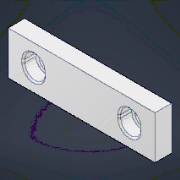
# Autodesk Inventor part: JawDualSided
Saved by Autodesk Inventor 2024.3 (Build 283343000, 343)
## iProperties
IsCustomPart: 1
Created: 2024-02-05
Part Number: JawDualSided
Material: Aluminum 6061
Document SubType Name: Modeling
Designer: fablabadmin
Language: en-US
Size Designation: JawDualSided-Aluminum 6061
Categories: <MemberInstance><Categories><Category DisplayName="CAM_JAWS" InternalName="a455355c-d78b-4130-92af-7f17fb1dc89c" Mnemonic="CAM_JAWS"/><Category DisplayName="DataType" InternalName="23b78d0f-2648-40c6-8793-ca6db495c9e8" Mnemonic="DATATYPE"><CategoryParameter DisplayName="DisplayName" InternalName="05415f3d-3907-474b-a020-eb9d644f4cf3" Mnemonic="DISPLAYNAME"/><CategoryParameter DisplayName="Standard" InternalName="0c0a119c-1e12-4c84-803f-101930972f5e" Mnemonic="STANDARD"/><CategoryParameter DisplayName="Description" InternalName="13903e3d-64b1-4950-80da-f627842ea37f" Mnemonic="DESCRIPTION"/><CategoryParameter DisplayName="Designation" InternalName="2675968c-4ce5-49e0-a4f5-552d29089031" Mnemonic="DESIGNATION"/><CategoryParameter DisplayName="Default Row" InternalName="2af9ec52-faaa-4026-b378-f9fa4afca842" Mnemonic="DEFAULTROW"/><CategoryParameter DisplayName="Folder Name" InternalName="3f06958e-8713-4116-9be7-ed6184ecc97b" Mnemonic="FOLDERNAME"/><CategoryParameter DisplayName="Revision Guid" InternalName="45a75005-10b1-4dfc-8d6d-dfe629f0b93c" Mnemonic="REVISIONGUID"/><CategoryParameter DisplayName="FileName" InternalName="8b46a4cc-9585-4fed-90c3-899f57e09a73" Mnemonic="FILENAME"/><CategoryParameter DisplayName="StdsOrg" InternalName="8f5914e1-4693-403f-8ab5-d37768198c9d" Mnemonic="STDSORG"/><CategoryParameter DisplayName="Family Version" InternalName="914462f6-6e19-4b14-ba84-155b9680b1d0" Mnemonic="FAMILYREVISION"/><CategoryParameter DisplayName="Standard Revision" InternalName="91d5a463-65c2-4fde-b823-3b7fea5e8e17" Mnemonic="STANDARDREVISION"/><CategoryParameter DisplayName="Member Revision" InternalName="a65d44b9-392f-4f4f-857b-e4b3d54996fe" Mnemonic="MEMBERREVISION"/><CategoryParameter DisplayName="ClipFormat" InternalName="bc51e27b-3422-4e78-93ef-cec197ddf230" Mnemonic="CLIPFORMAT"/><CategoryParameter DisplayName="Manufacturer" InternalName="cd6c7a72-a28a-4e50-99a9-2c7f4e13e5ad" Mnemonic="MANUFACTURER"/><CategoryParameter DisplayName="InternalName" InternalName="cf1d0246-76d9-4b4a-8305-fa0409afb5c1" Mnemonic="INTERNALNAME"/><CategoryParameter DisplayName="IsMetric" InternalName="e2385c5b-1ea4-4823-96a8-8de651266ec3" Mnemonic="ISMETRIC"/><Category DisplayName="Part" InternalName="c0e0b642-3bcb-4cc8-9e80-f96d35c4afa4" Mnemonic="PART"><CategoryParameter DisplayName="Part Number" InternalName="016b6077-bfbe-49bd-92c9-d8d59c39c941" Mnemonic="PARTNUMBER"/><CategoryParameter DisplayName="Stock Number" InternalName="4dba7c1c-e26c-444e-836c-b08b433409a8" Mnemonic="STOCKNUMBER"/><CategoryParameter DisplayName="Material Key" InternalName="5c9a8adb-dd2b-4535-b97f-0a94a95fe41f" Mnemonic="MATERIALKEY"/><CategoryParameter DisplayName="Material" InternalName="818a152a-d3c3-49ca-80ee-df7d91421b8e" Mnemonic="MATERIAL"/></Category></Category></Categories><FamilyTemplate Id="DualSidedJaw"><FamilyTemplateParameters><FamilyTemplateParameter ObjectType="kPartComponentDefinitionObject" ValueType="xs:string" Id="11" SubObjectId="Material"/><FamilyTemplateParameter ObjectType="kPropertyObject" ValueType="xs:string" Id="18" ObjectReferenceKey="{32853F0F-3444-11d1-9E93-0060B03C1CA6}" SubObjectId="5"/><FamilyTemplateParameter ObjectType="kPropertyObject" ValueType="xs:string" Id="19" ObjectReferenceKey="{32853F0F-3444-11d1-9E93-0060B03C1CA6}" SubObjectId="52"/></FamilyTemplateParameters></FamilyTemplate><CategoryParameterMap><ParamToTemplateMap><ParamToTemplate CategoryParameter="//CategoryParameter[@InternalName='cf1d0246-76d9-4b4a-8305-fa0409afb5c1']" ConstantValue="43a365f2-93b3-4b52-b820-3dbb13a23e22"/><ParamToTemplate CategoryParameter="//CategoryParameter[@InternalName='45a75005-10b1-4dfc-8d6d-dfe629f0b93c']" ConstantValue="9f47d84c-379b-4d57-88d0-f6fbd2db50da"/><ParamToTemplate CategoryParameter="//CategoryParameter[@InternalName='3f06958e-8713-4116-9be7-ed6184ecc97b']" ConstantValue="DualSidedJaw"/><ParamToTemplate CategoryParameter="//CategoryParameter[@InternalName='8f5914e1-4693-403f-8ab5-d37768198c9d']" TemplateParameter="5"/><ParamToTemplate CategoryParameter="//CategoryParameter[@InternalName='0c0a119c-1e12-4c84-803f-101930972f5e']" TemplateParameter="6"/><ParamToTemplate CategoryParameter="//CategoryParameter[@InternalName='91d5a463-65c2-4fde-b823-3b7fea5e8e17']" TemplateParameter="7"/><ParamToTemplate CategoryParameter="//CategoryParameter[@InternalName='cd6c7a72-a28a-4e50-99a9-2c7f4e13e5ad']" TemplateParameter="8"/><ParamToTemplate CategoryParameter="//CategoryParameter[@InternalName='13903e3d-64b1-4950-80da-f627842ea37f']" TemplateParameter="10"/><ParamToTemplate CategoryParameter="//CategoryParameter[@InternalName='05415f3d-3907-474b-a020-eb9d644f4cf3']" ConstantValue="JawDual"/><ParamToTemplate CategoryParameter="//CategoryParameter[@InternalName='914462f6-6e19-4b14-ba84-155b9680b1d0']" ConstantValue="11"/><ParamToTemplate CategoryParameter="//CategoryParameter[@InternalName='bc51e27b-3422-4e78-93ef-cec197ddf230']" ConstantValue="CF_INVENTOR.STDPARTS"/><ParamToTemplate CategoryParameter="//CategoryParameter[@InternalName='e2385c5b-1ea4-4823-96a8-8de651266ec3']" ConstantValue="true"/><ParamToTemplate CategoryParameter="//CategoryParameter[@InternalName='2af9ec52-faaa-4026-b378-f9fa4afca842']" ConstantValue="1"/><ParamToTemplate CategoryParameter="//CategoryParameter[@InternalName='8b46a4cc-9585-4fed-90c3-899f57e09a73']" ConstantValue="JawDualSided-Aluminum 6061"/><ParamToTemplate CategoryParameter="//CategoryParameter[@InternalName='a65d44b9-392f-4f4f-857b-e4b3d54996fe']" ConstantValue="5ccd6349-9766-45ff-ba35-29068830a0fb"/><ParamToTemplate CategoryParameter="//CategoryParameter[@InternalName='a65d44b9-392f-4f4f-857b-e4b3d54996fe']" ConstantValue="5ccd6349-9766-45ff-ba35-29068830a0fb"/><ParamToTemplate CategoryParameter="//CategoryParameter[@InternalName='2675968c-4ce5-49e0-a4f5-552d29089031']" TemplateParameter="19"/><ParamToTemplate CategoryParameter="//CategoryParameter[@InternalName='818a152a-d3c3-49ca-80ee-df7d91421b8e']" TemplateParameter="11"/><ParamToTemplate CategoryParameter="//CategoryParameter[@InternalName='016b6077-bfbe-49bd-92c9-d8d59c39c941']" TemplateParameter="18"/></ParamToTemplateMap></CategoryParameterMap></MemberInstance>
Density: 2.7 g/cm^3
Appearance: Aluminum - Flat
Author: fablabadmin
Autodesk Inventor part; units mm, degrees
ref_plane "YZ Plane" through (0, 0, 0) normal (1, 0, 0) x (0, 1, 0)
ref_plane "XZ Plane" through (0, 0, 0) normal (0, 1, 0) x (-1, 0, 0)
ref_plane "XY Plane" through (0, 0, 0) normal (0, 0, 1) x (1, 0, 0)
sketch "Sketch1" plane through (0, 0, 0) normal (0, 0, 1) x (1, 0, 0)
  line L0 (-105.56, 0) -> (105.56, 0) construction
  line L1 (0, -31.15) -> (0, 31.15) construction
  line L2 (-75.5, 22.25) -> (75.5, 22.25)
  line L3 (75.5, 22.25) -> (75.5, -22.25)
  line L4 (75.5, -22.25) -> (-75.5, -22.25)
  line L5 (-75.5, -22.25) -> (-75.5, 22.25)
  line L6 (-49.21, 1.55) -> (-49.21, -1.55) construction
  line L7 (-56.21, 1.55) -> (-56.21, -1.55)
  line L8 (-42.21, -1.55) -> (-42.21, 1.55)
  arc A0 (-42.21, 1.55) -> (-56.21, 1.55) centre (-49.21, 1.55) ccw
  arc A1 (-56.21, -1.55) -> (-42.21, -1.55) centre (-49.21, -1.55) ccw
  line L9 (49.21, 1.55) -> (49.21, -1.55) construction
  line L10 (56.21, 1.55) -> (56.21, -1.55)
  line L11 (42.21, -1.55) -> (42.21, 1.55)
  arc A2 (56.21, 1.55) -> (42.21, 1.55) centre (49.21, 1.55) ccw
  arc A3 (42.21, -1.55) -> (56.21, -1.55) centre (49.21, -1.55) ccw
  line L12 (-49.21, 1.55) -> (-49.21, -1.55) construction
  line L13 (-59.71, 1.55) -> (-59.71, -1.55)
  line L14 (-38.71, -1.55) -> (-38.71, 1.55)
  arc A4 (-38.71, 1.55) -> (-59.71, 1.55) centre (-49.21, 1.55) ccw
  arc A5 (-59.71, -1.55) -> (-38.71, -1.55) centre (-49.21, -1.55) ccw
  line L15 (59.71, 1.55) -> (59.71, -1.55)
  line L16 (38.71, -1.55) -> (38.71, 1.55)
  arc A6 (59.71, 1.55) -> (38.71, 1.55) centre (49.21, 1.55) ccw
  arc A7 (38.71, -1.55) -> (59.71, -1.55) centre (49.21, -1.55) ccw
  point P0 (0, 0)
  point P1 (-49.21, 0)
  point P2 (49.21, 0)
  point P3 (-49.21, 0)
  dimension "d0" = 44.5
  dimension "d1" = 151
  dimension "d26" = 14
  dimension "d27" = 20.7
  dimension "d28" = 98.42
  dimension "d29" = 21
  dimension "d30" = 1.55
  constraints: 36 end point, 16 point on circle, 11 symmetric about line, 8 centre point, 8 tangent, 5 equal length, 2 midpoint, 1 horizontal, 1 perpendicular, 1 point on line, 1 vertical, 6 other
  measures "d0" distance of L2.end L3.end
  measures "d1" distance of L2.start L2.end
  measures "d26" distance between parallel lines of L8 L7
  measures "d27" distance from line of L4 L6.end
  measures "d28" distance between parallel lines of L9 L6
  measures "d29" distance between parallel lines of L13 L14
  measures "d30" distance from line of L0 L6.end
extrude "Extrusion1" add sketch "Sketch1" against normal blind 18 contours L2 L3 L4 L5 | A0 L8 A1 L7 | L10 A3 L11 A2 | A4 L14 A5 L13 | L15 A7 L16 A6
extrude "Extrusion2" cut sketch "Sketch1" against normal through all contours A0 L8 A1 L7 | L10 A3 L11 A2
extrude "Extrusion3" cut sketch "Sketch1" against normal blind 12.78 contours L10 A3 L11 A2 | A4 L14 A5 L13 | L15 A7 L16 A6
chamfer "Chamfer3" distance 1 angle 45 4 edges at (0, 22.25, -18) (-75.5, 0, -18) (0, -22.25, -18) (75.5, 0, -18)
chamfer "Chamfer4" distance 1.5 angle 45 8 edges at (-49.21, 12.05, 0) (-38.71, 0, 0) (-49.21, -12.05, 0) (-59.71, 0, 0) (49.21, 12.05, 0) (59.71, 0, 0) (49.21, -12.05, 0) (38.71, 0, 0)
chamfer "Chamfer5" distance 0.5 angle 45 8 edges at (-49.21, 8.55, -18) (-56.21, 0, -18) (-49.21, -8.55, -18) (-42.21, 0, -18) (49.21, -8.55, -18) (56.21, 0, -18) (49.21, 8.55, -18) (42.21, 0, -18)
sketch "Sketch2" plane through (-75.5, 22.25, 0) normal (0, 1, 0) x (1, 0, 0)
  line L0 (0, 17) -> (151, 17) construction
  line L1 (0, 0) -> (0, 17) construction
  line L2 (151, 0) -> (0, 0) projected
  line L3 (151, 0) -> (151, 17) construction
  line L4 (75.5, 21.6) -> (75.5, -3.6) construction
  circle A0 centre (75.5, -32.1751) radius 47.5 construction
  line L5 (150, 18) -> (1, 18) projected
  line L6 (58.5, 18) -> (40.5, 0)
  line L7 (92.5, 18) -> (110.5, 0)
  line L8 (14.29, 0) -> (38.29, 0) projected
  line L9 (33, 0) -> (51, 18)
  line L10 (118, 0) -> (100, 18)
  circle A1 centre (75.5, -28.2107) radius 50 construction
  line L11 (56.5, 16) -> (94.5, 16)
  dimension "d54" = 95
  dimension "d57" = 45
  dimension "d59" = 70
  dimension "d60" = 45
  dimension "d61" = 85
  dimension "d62" = 100
  dimension "d68" = 2
  constraints: 10 end point, 8 point on line, 4 symmetric about line, 2 centre point, 2 tangent, 1 parallel
  measures "d54" diameter of A0
  measures "d57" angle of L2 L6
  measures "d59" distance of L7.end L6.end
  measures "d60" angle of L2 L9
  measures "d61" distance of L10.start L9.start
  measures "d62" diameter of A1
  measures "d68" distance between parallel lines of L5 L11
extrude "Extrusion6" cut sketch "Sketch2" against normal blind 35 contours L2 L6 L11 L7
extrude "Extrusion7" cut sketch "Sketch2" against normal blind 6 contours L2 L7 L5 L10 | L2 L9 L5 L6 | L11 L6 L5 L7
fillet "Fillet1" radius 10 2 edges at (-19, 1.75, -16) (19, 1.75, -16)
equation "\"d0\" = jawH"
equation "\"d1\" = jawW"
equation "\"d4\" = jawT"
equation "\"jawH\" = 44.5"
equation "\"jawW\" = 151"
equation "\"jawT\" = 18"
body "Solid1"
